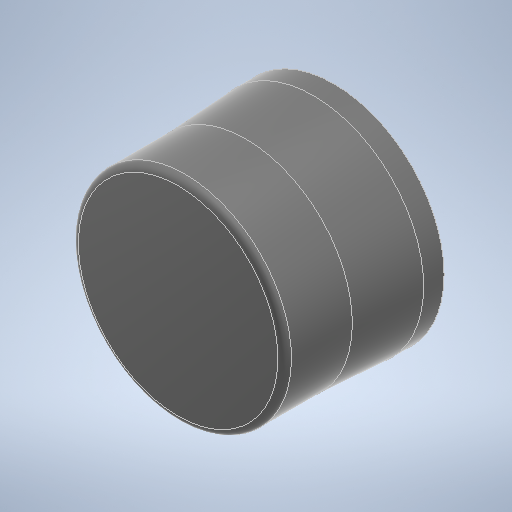
# Autodesk Inventor part: Spring_Top_2
Saved by Autodesk Inventor 2025.1 (Build 291241020, 241B)
## iProperties
Created: 2024-11-13
Part Number: Spring_Top_2
Material: PC/ABS Plastic
Document SubType Name: Modeling
Designer: leon-
Density: 1.1 g/cm^3
Appearance: Smooth - Black
Author: leon-
## iProperties of the stored document Spring_Top_3DPrint.ipt
Created: 2024-11-16
Part Number: Spring_Top_3DPrint
Material: Generic
Document SubType Name: Modeling
Designer: leon-
Density: 1 g/cm^3
Appearance: Default
Author: leon-
Autodesk Inventor part; units mm, degrees
ref_plane "YZ Plane" through (0, 0, 0) normal (1, 0, 0) x (0, 1, 0)
ref_plane "XZ Plane" through (0, 0, 0) normal (0, 1, 0) x (-1, 0, 0)
ref_plane "XY Plane" through (0, 0, 0) normal (0, 0, 1) x (1, 0, 0)
sketch "Sketch1" plane through (0, 0, 0) normal (1, 0, 0) x (0, 1, 0)
  line L0 (0, 0) -> (15.75, 0)
  line L1 (15.75, 0) -> (15.75, -10)
  line L2 (15.75, -10) -> (10.2, -10)
  line L3 (10.2, -10) -> (10.2, -5)
  line L4 (10.2, -5) -> (0, -5)
  line L5 (0, -5) -> (0, 0)
  point P0 (0, -2.5)
  point P1 (15.75, -5)
  point P2 (7.875, 0)
  dimension "d0" = 15.75
  dimension "d1" = 10.2
  dimension "d2" = 10
  dimension "d3" = 5
  constraints: 12 end point, 5 perpendicular, 3 midpoint, 1 horizontal
  measures "d0" horizontal distance of point (0, -2.5) point (15.75, -5)
  measures "d1" distance between parallel lines of L5 L3
  measures "d2" distance between parallel lines of L0 L2
  measures "d3" distance from line of point (7.875, 0) L4
revolve "Revolution1" add sketch "Sketch1" angle 360 about axis through (0, 0, -5) along (0, 0, 1)
sketch "Sketch3" plane through (0, 0, 0) normal (1, 0, 0) x (0, 1, 0)
  line L0 (15.75, 0) -> (-15.75, 0) projected
  line L1 (15.75, -10) -> (-15.75, -10) projected
  line L2 (15.75, -10) -> (15.75, 0) projected
  line L3 (15.75, -10) -> (16.3, -20)
  line L4 (15.5, -20.022) -> (14.9488, -10)
  line L5 (14.9488, -10) -> (15.75, -10)
  line L6 (0, -24.0479) -> (0, 4.008) projected
  line L7 (16.3, -20) -> (16.3, -23.022)
  line L8 (16.3, -23.022) -> (15.5, -23.022)
  line L9 (15.5, -23.022) -> (15.5, -20.022)
  point P0 (0, 0)
  point P1 (0, 0)
  dimension "d14" = 0.8
  dimension "d15" = 16.3
  dimension "d16" = 10
  dimension "d18" = 3
  dimension "d19" = 0.8
  constraints: 12 end point, 2 perpendicular, 1 collinear, 1 horizontal, 1 midpoint
  measures "d14" distance between parallel lines of L3 L4
  measures "d15" horizontal distance of point (0, 0) L3.end
  measures "d16" distance from line of L1 L3.end
  measures "d18" distance from line of L4.start L8
  measures "d19" distance between parallel lines of L7 L9
revolve "Revolution2" add sketch "Sketch3" angle 360 about axis through (0, 0, -10) along (0, 0, 1) contours L3 L7 L8 L9 L4 L1
fillet "Fillet2" radius 1 1 edges at (0, -15.75, 0)
body "Solid1"
